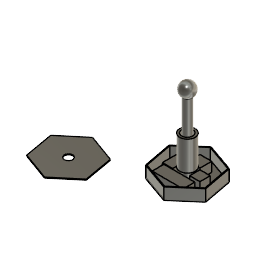
Tesla coil design (Autodesk Fusion 360 design; units mm, degrees)
Autodesk Fusion 360 part; units mm, degrees
sketch "Sketch5" plane through (0, 0, 0) normal (0, 0, 1) x (1, 0, 0)
  line L0 (70, -70) -> (-70, -70)
  line L1 (-70, -70) -> (-70, 70)
  line L2 (-70, 70) -> (70, 70)
  line L3 (70, 70) -> (70, -70)
  line L4 (70, -70) -> (-70, 70) construction
  line L5 (-70, -70) -> (70, 70) construction
  dimension "d13" = 140
  dimension "d14" = 140
  constraint horizontal L0
  constraint perpendicular L0 L1
  constraint parallel L0 L2
  constraint parallel L1 L3
  constraint coincident L4 origin
  constraint coincident L5 origin
  measures "d13" distance of L1.end L2.end
  measures "d14" distance of L0.end L1.end
extrude "Extrude3" add sketch "Sketch5" along normal blind 140 makes body 1
sketch "Sketch6" plane through (0, 0, 0) normal (0, 0, 1) x (1, 0, 0)
  line L0 (80, -80) -> (-80, -80)
  line L1 (-80, -80) -> (-80, 80)
  line L2 (-80, 80) -> (80, 80)
  line L3 (80, 80) -> (80, -80)
  line L4 (80, -80) -> (-80, 80) construction
  line L5 (-80, -80) -> (80, 80) construction
  dimension "d17" = 160
  dimension "d18" = 160
  constraint horizontal L0
  constraint perpendicular L0 L1
  constraint parallel L0 L2
  constraint parallel L1 L3
  constraint coincident L4 origin
  constraint coincident L5 origin
  measures "d17" distance of L1.end L2.end
  measures "d18" distance of L0.end L1.end
extrude "Extrude4" add sketch "Sketch6" along normal blind 140 separate body makes body 2
sketch "Sketch7" plane through (0, 0, 0) normal (0, 0, 1) x (1, 0, 0)
  line L0 (210, -80) -> (-210, -80)
  line L1 (-210, -80) -> (-210, 80)
  line L2 (-210, 80) -> (210, 80)
  line L3 (210, 80) -> (210, -80)
  line L4 (210, -80) -> (-210, 80) construction
  line L5 (-210, -80) -> (210, 80) construction
  dimension "d21" = 420
  dimension "d22" = 160
  constraint horizontal L0
  constraint perpendicular L0 L1
  constraint parallel L0 L2
  constraint parallel L1 L3
  constraint coincident L4 origin
  constraint coincident L5 origin
  measures "d21" distance of L1.end L2.end
  measures "d22" distance of L0.end L1.end
extrude "Extrude5" add sketch "Sketch7" along normal blind 140 separate body makes body 3
sketch "Sketch8" plane through (0, 0, 0) normal (0, 0, 1) x (1, 0, 0)
  line L0 (70, -100) -> (-70, -100)
  line L1 (-70, -100) -> (-70, 100)
  line L2 (-70, 100) -> (70, 100)
  line L3 (70, 100) -> (70, -100)
  line L4 (70, -100) -> (-70, 100) construction
  line L5 (-70, -100) -> (70, 100) construction
  dimension "d25" = 140
  dimension "d26" = 200
  constraint horizontal L0
  constraint perpendicular L0 L1
  constraint parallel L0 L2
  constraint parallel L1 L3
  constraint coincident L4 origin
  constraint coincident L5 origin
  measures "d25" distance of L1.end L2.end
  measures "d26" distance of L0.end L1.end
extrude "Extrude6" add sketch "Sketch8" along normal blind 140 separate body makes body 4
sketch "Sketch9" plane through (0, 0, 0) normal (0, 0, 1) x (1, 0, 0)
  circle A0 centre (0, 0) radius 57.5
  dimension "d29" = 115
  constraint coincident A0.centre origin
  measures "d29" diameter of A0
extrude "Extrude7" add sketch "Sketch9" along normal blind 1000 separate body makes body 5
hole "Hole1" at (0, 0, 1000) direction (0, 0, -1) diameter 100 depth 1000 tip angle 118 bodies 5
sphere "SpherePrimitive1" add diameter 200 placed x (1, 0, 0) y (0, 1, 0) z (0, 0, 1) at (0, 0, 0) separate body makes body 6
sketch "Sketch11" plane through (0, 0, 0) normal (0, 0, 1) x (1, 0, 0)
  circle A0 centre (0, 0) radius 105
  dimension "d36" = 210
  constraint coincident A0.centre origin
  measures "d36" diameter of A0
extrude "Extrude8" add sketch "Sketch11" along normal blind 400 separate body makes body 7
hole "Hole2" at (-2.019, -1.1373, 400) direction (0, 0, -1) diameter 150 depth 400 tip angle 118 bodies 7
move_body "Move1" bodies 7 to x (1, 0, 0) y (0, 1, 0) z (0, 0, 1) at (0, 0, 140)
move_body "Move2" bodies 2 to x (1, 0, 0) y (0, 1, 0) z (0, 0, 1) at (0, 170, 0)
move_body "Move3" bodies 6 to x (1, 0, 0) y (0, 1, 0) z (0, 0, 1) at (0, 0, 1100)
move_body "Move4" bodies 6 to x (1, 0, 0) y (0, 1, 0) z (0, 0, 1) at (0, 0, -25)
move_body "Move5" bodies 4 to x (1, 0, 0) y (0, 1, 0) z (0, 0, 1) at (-170, 0, 0)
move_body "Move6" bodies 1 to x (1, 0, 0) y (0, 1, 0) z (0, 0, 1) at (170, 0, 0)
move_body "Move7" bodies 3 to x (1, 0, 0) y (0, 1, 0) z (0, 0, 1) at (0, -180, 0)
move_body "Move8" bodies 3 to x (1, 0, 0) y (0, 1, 0) z (0, 0, 1) at (0, -10, 0)
move_body "Move9" bodies 7 to x (1, 0, 0) y (0, 1, 0) z (0, 0, 1) at (0, 0, 20)
sketch "Sketch12" plane through (0, 0, 0) normal (0, 0, 1) x (1, 0, 0)
  line L0 (415.6853, 2.394) -> (205.7694, 361.191)
  line L1 (205.7694, 361.191) -> (-209.9159, 358.7971)
  line L2 (-209.9159, 358.7971) -> (-415.6853, -2.394)
  line L3 (-415.6853, -2.394) -> (-205.7694, -361.191)
  line L4 (-205.7694, -361.191) -> (209.9159, -358.7971)
  line L5 (209.9159, -358.7971) -> (415.6853, 2.394)
  dimension "d42" = 360
  measures "d42" distance of origin L5
extrude "Extrude9" cut sketch "Sketch12" along normal blind 10 bodies 1 2 3 4
sketch "Sketch13" plane through (0, 0, 0) normal (0, 0, 1) x (1, 0, 0)
  line L0 (381.5229, -133.3176) -> (306.2179, 263.7497)
  line L1 (306.2179, 263.7497) -> (-75.305, 397.0674)
  line L2 (-75.305, 397.0674) -> (-381.5229, 133.3176)
  line L3 (-381.5229, 133.3176) -> (-306.2179, -263.7497)
  line L4 (-306.2179, -263.7497) -> (75.305, -397.0674)
  line L5 (75.305, -397.0674) -> (381.5229, -133.3176)
  dimension "d45" = 350
  measures "d45" distance of origin L5
extrude "Extrude10" add sketch "Sketch13" along normal blind 160 separate body makes body 8
shell "Shell1" thickness 12 removed faces 1 at (127.1743, -44.4392, 160) on bodies 8
sketch "Sketch16" plane through (0, 0, 0) normal (0, 0, 1) x (1, 0, 0)
  line L0 (-202.0726, 350) -> (-404.1452, 0)
  line L1 (-404.1452, 0) -> (-202.0726, -350)
  line L2 (-202.0726, -350) -> (202.0726, -350)
  line L3 (202.0726, -350) -> (404.1452, 0)
  line L4 (404.1452, 0) -> (202.0726, 350)
  line L5 (202.0726, 350) -> (-202.0726, 350)
  circle A0 centre (0, 0) radius 56
  dimension "d49" = 350
  dimension "d50" = 112
  constraint coincident A0.centre origin
  measures "d49" distance of A0.centre L5
  measures "d50" diameter of A0
extrude "Extrude11" add sketch "Sketch16" along normal blind 12 separate body makes body 9
move_body "Move10" bodies 9 to x (0.422618, 0.906308, 0) y (-0.906308, 0.422618, 0) z (0, 0, 1) at (-23.7075, -1764.1746, 0)
move_body "Move11" bodies 9 to x (0.819152, 0.573576, 0) y (-0.573576, 0.819152, 0) z (0, 0, 1) at (-881.3889, 1481.5214, 0)
move_body "Move12" bodies 9 to x (1, 0, 0) y (0, 1, 0) z (0, 0, 1) at (0, 0, 200)
move_body "Move13" bodies 9 to x (1, 0, 0) y (0, 1, 0) z (0, 0, 1) at (-100, 0, 0)
move_body "Move14" bodies 9 to x (1, 0, 0) y (0, 1, 0) z (0, 0, 1) at (0, -31, 0)
move_body "Move15" bodies 9 to x (1, 0, 0) y (0, 1, 0) z (0, 0, 1) at (-880.9511, -739.2058, 0)
equation "d29 = 110 mm + 5 mm"
equation "d46 = 140 mm + 20 mm"
equation "d50 = 110 mm + 2 mm"
named bodies: "SparkGap", "CapBox", "MOT Box", "Aduino Unit", "SecondaryCoil", "TopLoad", "PrimaryCoil"
